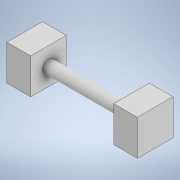
# Autodesk Inventor part: belt axle
Saved by Autodesk Inventor 2020 (Build 240168000, 168)
## iProperties
Created: 2021-07-04
Part Number: belt axle
Material: Generic
Document SubType Name: Modeling
Designer: pc
Density: 1 g/cm^3
Appearance: Default
Author: pc
Autodesk Inventor part; units mm, degrees
ref_plane "YZ Plane" through (0, 0, 0) normal (1, 0, 0) x (0, 1, 0)
ref_plane "XZ Plane" through (0, 0, 0) normal (0, 1, 0) x (-1, 0, 0)
ref_plane "XY Plane" through (0, 0, 0) normal (0, 0, 1) x (1, 0, 0)
sketch "Sketch1" plane through (0, 0, 0) normal (1, 0, 0) x (0, 1, 0)
  line L0 (9.0933, 11.7239) -> (-29.0067, 11.7239)
  line L1 (-29.0067, 11.7239) -> (-29.0067, -26.3761)
  line L2 (-29.0067, -26.3761) -> (9.0933, -26.3761)
  line L3 (9.0933, -26.3761) -> (9.0933, 11.7239)
  circle A0 centre (-9.9567, -7.3261) radius 6.35
  point P0 (0, 0)
  dimension "d0" = 38.1
  dimension "d1" = 38.1
  dimension "d2" = 12.7
  dimension "d3" = 19.05
  dimension "d4" = 19.05
  constraints: 8 end point, 2 parallel, 1 centre point, 1 horizontal, 1 perpendicular
  measures "d0" distance of L2.end L1.end
  measures "d1" distance of L1.end L0.end
  measures "d2" diameter of A0
  measures "d3" distance from line of A0.centre L3
  measures "d4" distance from line of L0 A0.centre
extrude "Extrusion1" add sketch "Sketch1" along normal blind 25.4 contours L3 L2 L1 L0 | A0
sketch "Sketch2" plane through (25.4, 0, 0) normal (1, 0, 0) x (0, 0, -1)
  circle A0 centre (7.3261, -9.9567) radius 6.35
  line L0 (-11.7239, 9.0933) -> (-11.7239, -29.0067) projected
  line L1 (26.3761, 9.0933) -> (-11.7239, 9.0933) projected
  point P0 (0, 0)
  dimension "d7" = 12.7
  dimension "d8" = 19.05
  dimension "d9" = 19.05
  constraints: 1 centre point
  measures "d7" diameter of A0
  measures "d8" distance from line of A0.centre L0
  measures "d9" distance from line of A0.centre L1
extrude "Extrusion2" add sketch "Sketch2" along normal blind 88.9
sketch "Sketch3" plane through (114.3, -9.9567, -7.3261) normal (1, 0, 0) x (0, 0, -1)
  line L0 (-18.9201, 19.115) -> (19.1799, 19.115)
  line L1 (19.1799, 19.115) -> (19.1799, -18.985)
  line L2 (19.1799, -18.985) -> (-18.9201, -18.985)
  line L3 (-18.9201, -18.985) -> (-18.9201, 19.115)
  point P0 (-7.3261, 9.9567)
  dimension "d12" = 38.1
  dimension "d13" = 38.1
  constraints: 8 end point, 2 parallel, 1 horizontal, 1 perpendicular
  measures "d12" distance of L1.end L2.end
  measures "d13" distance of L0.end L1.end
extrude "Extrusion3" add sketch "Sketch3" along normal blind 25.4
body "Solid1"
